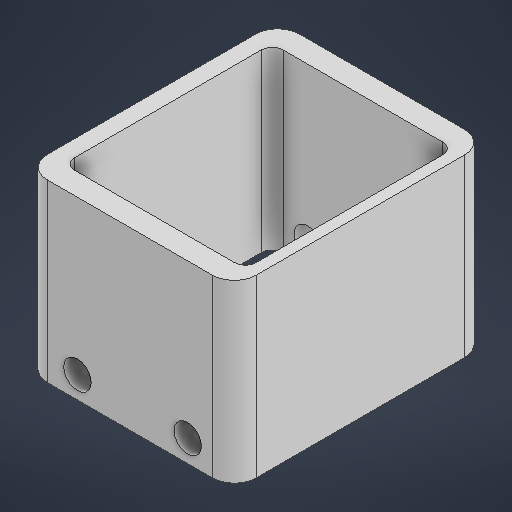
# Autodesk Inventor part: soporte inyector salida
Saved by Autodesk Inventor 2026.1 (Build 301233020, 233B)
## iProperties
Created: 2025-12-21
Part Number: soporte inyector salida
Material: Genérico
Document SubType Name: Modeling
Designer: patri
Density: 1 g/cm^3
Appearance: Valor por defecto
Author: patri
Autodesk Inventor part; units mm, degrees
ref_plane "YZ Plane" through (0, 0, 0) normal (1, 0, 0) x (0, 1, 0)
ref_plane "XZ Plane" through (0, 0, 0) normal (0, 1, 0) x (-1, 0, 0)
ref_plane "XY Plane" through (0, 0, 0) normal (0, 0, 1) x (1, 0, 0)
sketch "Boceto1" plane through (0, 0, 0) normal (0, 0, 1) x (1, 0, 0)
  line L0 (0, 0) -> (19.05, 0)
  line L1 (19.05, 0) -> (19.05, 16)
  line L2 (19.05, 16) -> (0, 16)
  line L3 (0, 16) -> (0, 0)
  circle A0 centre (14.8, 2) radius 1.25
  circle A1 centre (4.75, 2) radius 1.25
  line L4 (18.05, 0) -> (18.05, 16)
  line L5 (1.5, 0) -> (1.5, 16)
  dimension "d0" = 19.05
  dimension "d1" = 16
  dimension "d2" = 2.5
  dimension "d3" = 2.5
  dimension "d4" = 1
  dimension "d5" = 1.5
  dimension "d6" = 2
  dimension "d7" = 2
  dimension "d8" = 3.25
  dimension "d9" = 3.25
  constraints: 12 end point, 4 point on line, 2 centre point, 2 parallel, 2 perpendicular, 1 horizontal, 1 vertical
  measures "d0" distance of L2.end L1.end
  measures "d1" distance of L1.end L0.end
  measures "d2" diameter of A0
  measures "d3" diameter of A1
  measures "d4" distance between parallel lines of L1 L4
  measures "d5" distance between parallel lines of L5 L3
  measures "d6" distance from line of L0 A0.centre
  measures "d7" distance from line of L0 A1.centre
  measures "d8" distance from line of A1.centre L5
  measures "d9" distance from line of L4 A0.centre
extrude "Extrusión1" add sketch "Boceto1" along normal blind 23 contours L3 L2 L5 L0 | L4 L2 L1 L0
extrude "Extrusión2" add sketch "Boceto1" along normal blind 2 contours L5 L2 L4 L0
extrude "Extrusión3" add sketch "Boceto1" against normal blind 2 from surface at 23 contours L5 L2 L4 L0
fillet "Empalme1" radius 1 4 edges at (1.5, 8, 2) (18.05, 8, 2) (18.05, 8, 21) (1.5, 8, 21)
fillet "Empalme2" radius 2 4 edges at (19.05, 8, 23) (0, 8, 23) (0, 8, 0) (19.05, 8, 0)
equation "\"d2\" = d3"
